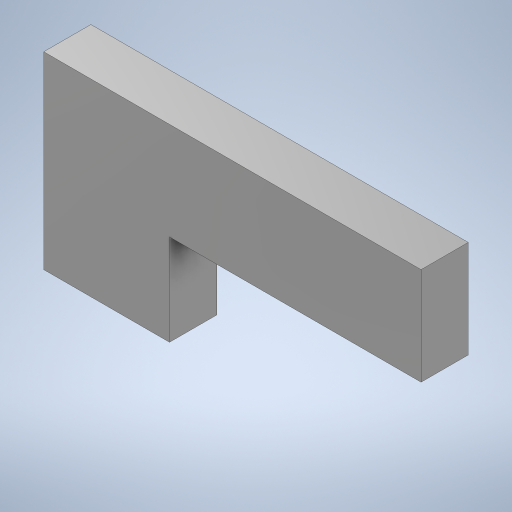
# Autodesk Inventor part: laser-enclosure
Saved by Autodesk Inventor 2023 (Build 270158000, 158)
## iProperties
Created: 2023-03-17
Part Number: laser-enclosure
Material: Generic
Document SubType Name: Modeling
Designer: kk4764
Density: 1 g/cm^3
Appearance: Default
Author: kk4764
Autodesk Inventor part; units mm, degrees
ref_plane "YZ Plane" through (0, 0, 0) normal (1, 0, 0) x (0, 1, 0)
ref_plane "XZ Plane" through (0, 0, 0) normal (0, 1, 0) x (-1, 0, 0)
ref_plane "XY Plane" through (0, 0, 0) normal (0, 0, 1) x (1, 0, 0)
sketch "Sketch1" plane through (0, 0, 0) normal (0, 0, 1) x (1, 0, 0)
  line L0 (0, 0) -> (1524, 0)
  line L1 (1524, 0) -> (1524, -393.7)
  line L2 (1524, -393.7) -> (508, -393.7)
  line L3 (0, -393.7) -> (0, 0)
  line L4 (0, 0) -> (928.4892, 0)
  line L5 (420.4892, -393.7) -> (508, -393.7)
  line L6 (0, -393.7) -> (0, 0)
  line L7 (0, 0) -> (508, 0)
  line L8 (508, -393.7) -> (508, -762)
  line L9 (508, -762) -> (0, -762)
  line L10 (0, -762) -> (0, 0)
  dimension "d0" = 393.7
  dimension "d1" = 1524
  dimension "d2" = 762
  dimension "d3" = 508
  constraints: 22 end point, 5 parallel, 3 horizontal, 2 perpendicular, 1 point on line
  measures "d0" distance of L0.end L1.end
  measures "d1" distance of L1.end L3.start
  measures "d2" distance of L7.end L8.end
  measures "d3" distance of L8.end L9.end
extrude "Extrusion1" add sketch "Sketch1" along normal blind 190.5
body "Solid1"
